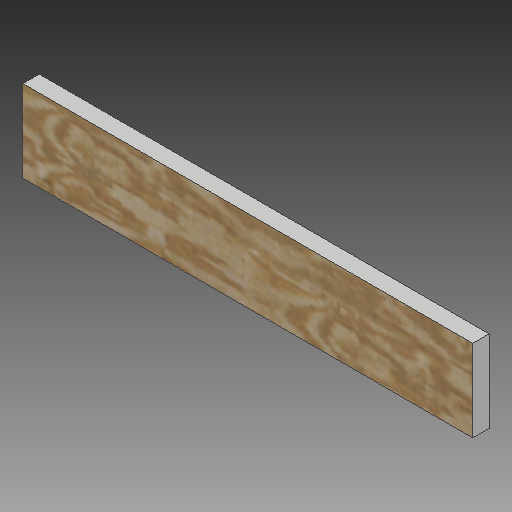
# Autodesk Inventor part: Wheel mounting side part
Saved by Autodesk Inventor 2018.2 (Build 222227000, 227)
## iProperties
Created: 2018-02-27
Part Number: Wheel mounting side part
Material: Generic
Document SubType Name: Modeling
Designer: owner
Density: 1 g/cm^3
Appearance: Default
Author: owner
Autodesk Inventor part; units mm, degrees
ref_plane "YZ Plane" through (0, 0, 0) normal (1, 0, 0) x (0, 1, 0)
ref_plane "XZ Plane" through (0, 0, 0) normal (0, 1, 0) x (-1, 0, 0)
ref_plane "XY Plane" through (0, 0, 0) normal (0, 0, 1) x (1, 0, 0)
sketch "Sketch1" plane through (0, 0, 0) normal (0, 0, 1) x (1, 0, 0)
  line L0 (-1015.3645, -325.5837) -> (-298.4241, -325.5837) projected
  line L1 (-298.4241, -325.5837) -> (-298.4241, -306.5337) projected
  line L2 (-298.4241, -306.5337) -> (-1015.3645, -306.5337) projected
  line L3 (-1015.3645, -306.5337) -> (-1015.3645, -325.5837) projected
  line L4 (-789.3945, -443.9607) -> (-694.1445, -443.9607) projected
  line L5 (-1015.3645, -325.5837) -> (-317.4741, -325.5837)
  line L6 (-317.4741, -452.5837) -> (-1015.3645, -452.5837)
  line L7 (-1015.3645, -452.5837) -> (-1015.3645, -325.5837)
  line L8 (-317.4741, -452.5837) -> (-317.4741, -325.5837)
  point P0 (0, 0)
  dimension "d2" = 716.9404
  dimension "d4" = 127
  constraints: 8 end point, 1 horizontal, 1 parallel, 1 perpendicular
  measures "d2" distance of L0.start L0.end
  measures "d4" distance of L6.start L5.end
extrude "Extrusion1" add sketch "Sketch1" along normal blind 25.4 contours L0 L8 L6 L7
body "Solid1"
